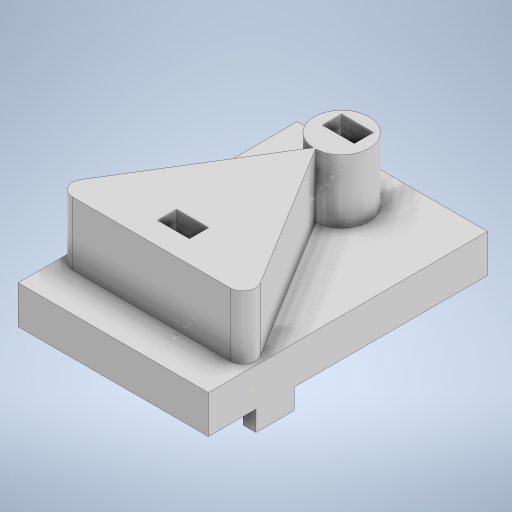
# Autodesk Inventor part: NOTGATE2
Saved by Autodesk Inventor 2024 (Build 280153000, 153)
## iProperties
Created: 2024-03-14
Part Number: NOTGATE2
Material: Generic
Document SubType Name: Modeling
Designer: Jonat
Density: 1 g/cm^3
Appearance: Default
Author: Jonat
Autodesk Inventor part; units mm, degrees
ref_plane "YZ Plane" through (0, 0, 0) normal (1, 0, 0) x (0, 1, 0)
ref_plane "XZ Plane" through (0, 0, 0) normal (0, 1, 0) x (-1, 0, 0)
ref_plane "XY Plane" through (0, 0, 0) normal (0, 0, 1) x (1, 0, 0)
sketch "Sketch5" plane through (0, 0, 0) normal (0, 1, 0) x (-1, 0, 0)
  line L0 (-3.1299, 16.302) -> (-3.1299, -27.8812) construction
  line L1 (-3.1299, -27.8812) -> (-19.0358, -27.8812) construction
  line L2 (-19.0358, -27.8812) -> (-19.0358, 16.302) construction
  line L3 (-19.0358, 16.302) -> (-3.1299, 16.302) construction
  line L4 (0, 0) -> (16, 0)
  line L5 (8, 0) -> (8, -24.9508) construction
  line L6 (16, 0) -> (8, -13)
  line L7 (8, -13) -> (0, 0)
  circle A0 centre (8, -15) radius 2.1568
  line L8 (0, 0) -> (0, -12.5098) construction
  point P0 (7.9048, -12.8453)
  point P1 (8.0952, -12.8453)
  dimension "d36" = 16
  dimension "d42" = 13
  dimension "d43" = 2
  constraints: 10 end point, 2 perpendicular, 2 point on line, 1 centre point, 1 horizontal, 1 midpoint, 1 parallel, 1 vertical, 2 other
  measures "d36" distance of L4.start L4.end
  measures "d42" distance from line of L4 L6.end
  measures "d43" distance of L6.end A0.centre
extrude "Extrusion4" add sketch "Sketch5" along normal blind 5
sketch "Sketch6" plane through (0, 5, 0) normal (0, 1, 0) x (1, 0, 0)
  arc A0 (-7.9048, 12.8453) -> (-8.0952, 12.8453) centre (-8, 15) ccw projected
  circle A1 centre (-8, 15) radius 1.6568
  line L0 (-16, 0) -> (0, 0) projected
  line L1 (-16, 0) -> (0, 0) construction
  line L2 (-14.2104, 1) -> (-8, 11.092)
  line L3 (-8.0952, 12.8453) -> (-16, 0) projected
  line L4 (-8, 11.092) -> (-1.7896, 1)
  line L5 (0, 0) -> (-7.9048, 12.8453) projected
  line L6 (-14.2104, 1) -> (-1.7896, 1)
  line L7 (-8, 15) -> (-8, 0) construction
  dimension "d46" = 0.5
  dimension "d52" = 1
  dimension "d53" = 1
  constraints: 10 end point, 3 parallel, 1 centre point, 1 coincident, 1 horizontal, 1 midpoint, 1 point on line
  measures "d46" radial gap between concentric circles of A0 A1
  measures "d52" distance between parallel lines of L0 L6
  measures "d53" distance between parallel lines of L3 L2
extrude "Extrusion5" [suppressed]
fillet "Fillet1" radius 1 2 edges at (0, 2.5, 0) (-16, 2.5, 0)
sketch "Sketch9" plane through (0, 0, 0) normal (0, -1, 0) x (1, 0, 0)
  line L0 (-15.5, 3) -> (-0.5, 3)
  line L1 (-0.5, 3) -> (-0.5, -19)
  line L2 (-0.5, -19) -> (-15.5, -19)
  line L3 (-15.5, -19) -> (-15.5, 3)
  line L4 (-15.5, 3) -> (-0.5, -19) construction
  line L5 (-0.5, 3) -> (-15.5, -19) construction
  line L6 (-14.2104, 0) -> (-1.7896, 0) projected
  line L7 (-8, -15) -> (-8, 0) construction
  arc A0 (-8.0952, -12.8453) -> (-7.9048, -12.8453) centre (-8, -15) ccw construction
  circle A1 centre (-8, -15) radius 2.1568 construction
  point P0 (0, 0)
  point P1 (-8, -8)
  dimension "d75" = 15
  dimension "d76" = 22
  dimension "d77" = 3
  constraints: 14 end point, 3 midpoint, 2 coincident, 2 parallel, 1 centre point, 1 horizontal, 1 perpendicular, 1 point on line
  measures "d75" distance of L1.end L2.end
  measures "d76" distance of L0.end L1.end
  measures "d77" distance between parallel lines of L6 L0
extrude "Extrusion7" add sketch "Sketch9" along normal blind 3
sketch "Sketch10" plane through (0, -3, 0) normal (0, -1, 0) x (1, 0, 0)
  line L0 (-0.5, -19) -> (-0.5, 3) projected
  line L1 (-0.5, -0.75) -> (-1.5, -0.75)
  line L2 (-1.5, -0.75) -> (-1.5, -3.75)
  line L3 (-1.5, -3.75) -> (-0.5, -3.75)
  line L4 (-0.5, -3.75) -> (-0.5, -0.75)
  line L5 (-15.5, 3) -> (-15.5, -19) projected
  line L6 (-15.5, -0.75) -> (-14.5, -0.75)
  line L7 (-14.5, -0.75) -> (-14.5, -3.75)
  line L8 (-14.5, -3.75) -> (-15.5, -3.75)
  line L9 (-15.5, -3.75) -> (-15.5, -0.75)
  line L10 (-0.5, 3) -> (-15.5, 3) projected
  point P0 (0, 0)
  point P1 (-15.5, -3.75)
  point P2 (-0.5, -3.75)
  dimension "d80" = 1
  dimension "d81" = 3
  dimension "d82" = 1
  dimension "d83" = 3
  dimension "d84" = 3.75
  dimension "d85" = 3.75
  constraints: 16 end point, 4 parallel, 2 horizontal, 2 perpendicular, 2 point on line
  measures "d80" distance of L3.end L2.end
  measures "d81" distance of L2.end L1.end
  measures "d82" distance of L7.end L8.end
  measures "d83" distance of L6.end L7.end
  measures "d84" distance between parallel lines of L10 L6
  measures "d85" distance between parallel lines of L10 L1
extrude "Extrusion8" add sketch "Sketch10" along normal blind 1.6
sketch "Sketch11" plane through (0, -3, 0) normal (0, -1, 0) x (1, 0, 0)
  line L0 (-9.25, -1.75) -> (-6.75, -1.75)
  line L1 (-6.75, -1.75) -> (-6.75, -3.25)
  line L2 (-6.75, -3.25) -> (-9.25, -3.25)
  line L3 (-9.25, -3.25) -> (-9.25, -1.75)
  line L4 (-8, 0) -> (-8, -15.1696) construction
  line L5 (-15.5, -19) -> (-0.5, -19) construction
  line L6 (-8, -19) -> (-8, 3) construction
  line L7 (-0.5, 3) -> (-15.5, 3) construction
  line L8 (-1.5, -0.75) -> (-1.5, -3.75) projected
  line L9 (-14.5, -3.75) -> (-14.5, -0.75) projected
  line L10 (-0.5, -0.75) -> (-1.5, -0.75) projected
  line L11 (-15.5, -3.75) -> (-15.5, -19) projected
  line L12 (-6.75, -14.75) -> (-9.25, -14.75)
  line L13 (-9.25, -14.75) -> (-9.25, -16.25)
  line L14 (-9.25, -16.25) -> (-6.75, -16.25)
  line L15 (-6.75, -16.25) -> (-6.75, -14.75)
  line L16 (-6.75, -14.75) -> (-9.25, -16.25) construction
  line L17 (-9.25, -14.75) -> (-6.75, -16.25) construction
  line L18 (-1.5, -3.75) -> (-0.5, -3.75) projected
  point P0 (0, 0)
  point P1 (-8, -1.75)
  point P2 (-9.25, -2.5)
  point P3 (-8, -3.25)
  point P4 (-8, 0)
  point P5 (-8, -8)
  point P6 (-6.75, -2.5)
  point P7 (-8, -15.5)
  point P8 (-6.75, -15.5)
  dimension "d129" = 7.5
  dimension "d133" = 1.5
  dimension "d136" = 2.5
  dimension "d137" = 1.5
  dimension "d138" = 13
  dimension "d141" = 0.5
  constraints: 24 end point, 10 midpoint, 5 parallel, 2 horizontal, 2 perpendicular, 1 point on line, 1 vertical
  measures "d129" distance between parallel lines of L11 L4
  measures "d133" distance of L2.end L0.start
  measures "d136" distance of L14.end L13.end
  measures "d137" distance of L13.end L12.end
  measures "d138" distance of point (-6.75, -15.5) point (-6.75, -2.5)
  measures "d141" distance between parallel lines of L18 L2
extrude "Extrusion9" cut sketch "Sketch11" against normal blind 16
sketch "Sketch13" plane through (0, -3, 0) normal (0, -1, 0) x (1, 0, 0)
  line L0 (-1.5, 2) -> (-14.5, 2)
  line L1 (-14.5, 2) -> (-14.5, -18)
  line L2 (-14.5, -18) -> (-1.5, -18)
  line L3 (-1.5, -18) -> (-1.5, 2)
  line L4 (-0.5, 3) -> (-15.5, 3) projected
  line L5 (-0.5, -0.75) -> (-0.5, 3) projected
  line L6 (-15.5, 3) -> (-15.5, -0.75) projected
  line L7 (-15.5, -19) -> (-0.5, -19) projected
  point P0 (0, 0)
  point P1 (-15.5, 1.125)
  dimension "d106" = 1
  dimension "d107" = 1
  dimension "d108" = 1
  dimension "d109" = 1
  constraints: 8 end point, 2 parallel, 1 horizontal, 1 midpoint, 1 perpendicular
  measures "d106" distance between parallel lines of L4 L0
  measures "d107" distance between parallel lines of L5 L3
  measures "d108" distance from line of point (-15.5, 1.125) L1
  measures "d109" distance between parallel lines of L7 L2
extrude "Extrusion11" cut sketch "Sketch13" against normal blind 2
sketch "Sketch14" plane through (0, -1, 0) normal (0, -1, 0) x (1, 0, 0)
  line L0 (-9.25, -14.75) -> (-9.25, -16.25) construction
  line L1 (-9.25, -15.5) -> (-6.75, -15.5) construction
  line L2 (-6.75, -16.25) -> (-6.75, -14.75) construction
  line L3 (-9.25, -16.25) -> (-6.75, -16.25) construction
  line L4 (-8, -16.25) -> (-8, -1.75) construction
  line L5 (-6.75, -1.75) -> (-9.25, -1.75) construction
  line L6 (-9.25, -1.75) -> (-9.25, -3.25) construction
  line L7 (-9.25, -2.5) -> (-6.75, -2.5) construction
  line L8 (-6.25, -16.25) -> (-9.75, -16.25)
  line L9 (-9.75, -16.25) -> (-9.75, -14.75)
  line L10 (-9.75, -14.75) -> (-6.25, -14.75)
  line L11 (-6.25, -14.75) -> (-6.25, -16.25)
  line L12 (-6.25, -16.25) -> (-9.75, -14.75) construction
  line L13 (-9.75, -16.25) -> (-6.25, -14.75) construction
  line L14 (-6.25, -1.75) -> (-9.75, -1.75)
  line L15 (-9.75, -1.75) -> (-9.75, -3.25)
  line L16 (-9.75, -3.25) -> (-6.25, -3.25)
  line L17 (-6.25, -3.25) -> (-6.25, -1.75)
  line L18 (-6.25, -1.75) -> (-9.75, -3.25) construction
  line L19 (-9.75, -1.75) -> (-6.25, -3.25) construction
  point P0 (0, 0)
  point P1 (-8, -15.5)
  point P2 (-8, -2.5)
  dimension "d139" = 3.5
  dimension "d140" = 1.5
  constraints: 30 end point, 11 midpoint, 4 parallel, 3 horizontal, 2 equal length, 2 perpendicular, 1 point on line
  measures "d139" distance of L9.end L10.end
  measures "d140" distance of L8.end L9.end
extrude "Extrusion12" cut sketch "Sketch14" against normal blind 1
sketch "Sketch15" plane through (0, -1, 0) normal (0, -1, 0) x (1, 0, 0)
  circle A0 centre (-8, -8.25) radius 1.25
  line L0 (-8, 0) -> (-8, -15) construction
  circle A1 centre (-8, -8.25) radius 1.95
  line L1 (-14.5, 2) -> (-1.5, 2) projected
  line L2 (-9.25, -3.25) -> (-6.75, -3.25) projected
  point P0 (0, 0)
  point P1 (-10.0959, -3.25)
  point P2 (-13.4041, -3.25)
  point P3 (-6.25, -3.25)
  point P4 (-9.75, -3.25)
  dimension "d117" = 2.5
  dimension "d118" = 0.7
  dimension "d131" = 10.25
  constraints: 2 centre point, 2 end point, 1 coincident, 1 point on line, 1 vertical
  measures "d117" diameter of A0
  measures "d118" radial gap between concentric circles of A0 A1
  measures "d131" distance from line of L1 A0.centre
extrude "Extrusion13" add sketch "Sketch15" along normal blind 2 contours A0 | A1
sketch "Sketch17" plane through (0, -1, 0) normal (0, -1, 0) x (1, 0, 0)
  point P0 (0, 0)
sketch "Sketch16" plane through (-8, -3, -8.25) normal (0, -1, 0) x (1, 0, 0)
  circle A0 centre (0, 0) radius 1.95 projected
  circle A1 centre (0, 0) radius 1.25
  point P0 (8, 8.25)
  point P1 (-1.9339, 0.25)
  point P2 (1.9339, 0.25)
  dimension "d123" = 2.5
  dimension "d60" = 2.5
  dimension "d61" = 0.7
  dimension "d62" = 2.5
  dimension "d63" = 1.5
  dimension "d68" = 13
  dimension "d69" = 3.75
  dimension "d70" = 3.75
  dimension "d72" = 3.75
  dimension "d0" = 15
  dimension "d2" = 10
  dimension "d11" = 5
  dimension "d12" = 1.8
  constraints: 1 centre point, 1 coincident
  measures "d123" diameter of A1
extrude "Extrusion14" cut sketch "Sketch16" against normal blind 5 contours A1
body "Solid3"
